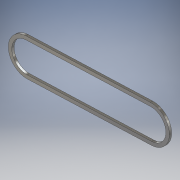
# Autodesk Inventor part: Chain
Saved by Autodesk Inventor 2017 (Build 210142000, 142)
## iProperties
Created: 2017-06-10
Part Number: Chain
Material: Generic
Document SubType Name: Modeling
Designer: Matthew
Density: 1 g/cm^3
Appearance: Chrome - Polished
Author: Matthew
Autodesk Inventor part; units mm, degrees
ref_plane "YZ Plane" through (0, 0, 0) normal (1, 0, 0) x (0, 1, 0)
ref_plane "XZ Plane" through (0, 0, 0) normal (0, 1, 0) x (-1, 0, 0)
ref_plane "XY Plane" through (0, 0, 0) normal (0, 0, 1) x (1, 0, 0)
sketch "Sketch1" plane through (0, 0, 0) normal (0, 0, 1) x (1, 0, 0)
  arc A0 (3.487, 25.0215) -> (1.7914, 25.1997) centre (0, 0) ccw
  arc A1 (5.6634, 19.703) -> (-1.4432, 20.4499) centre (0, 0) ccw
  arc A2 (164.4584, 30.6266) -> (162.8369, 30.0997) centre (171.45, 6.35) ccw
  arc A3 (168.6099, 26.6531) -> (161.8138, 24.4449) centre (171.45, 6.35) ccw
  arc A4 (172.385, -18.896) -> (170.515, 31.596) centre (171.45, 6.35) ccw
  arc A5 (172.2088, -14.1368) -> (170.6912, 26.8368) centre (171.45, 6.35) ccw
  arc A6 (-0.935, 25.246) -> (0.935, -25.246) centre (0, 0) ccw
  arc A7 (-0.7588, 20.4868) -> (0.7588, -20.4868) centre (0, 0) ccw
  line L0 (-0.935, 25.246) -> (170.515, 31.596)
  line L1 (0.935, -25.246) -> (172.385, -18.896)
  line L2 (-0.7588, 20.4868) -> (170.6912, 26.8368)
  line L3 (0.7588, -20.4868) -> (172.2088, -14.1368)
  point P0 (0, 0)
  constraints: 20 point on circle, 8 centre point, 8 end point, 8 tangent, 4 coincident
extrude "Extrusion1" add sketch "Sketch1" along normal blind 3.175
body "Solid1"
